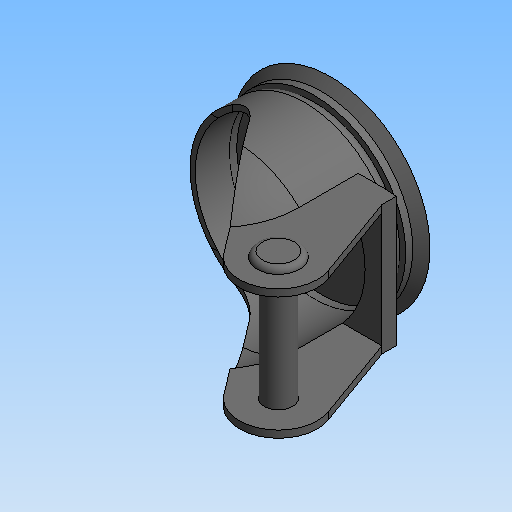
# Autodesk Inventor part: BODY-HSMCS50
Saved by Autodesk Inventor 2020 (Build 240168000, 168)
## iProperties
Part Number: BODY-HSMCS50
Material: 一般
Catalog Web Link: www.cadenas.de
Description: HSMC-BODY-Casters for Aluminum Frames-Corner Angle Type
Vendor: MISUMI
Document SubType Name: Modeling
Designer: partserver
Manufacturer: MISUMI
Mass: 15.0578 g
Surface Area: 150.838 cm^2
Volume: 15.0578 cm^3
Density: 1 g/cm^3
Appearance: PSOLRGB-128-128-128
Category: PARTsolutions
Company: MISUMI
PSOL_IDENT_0: {$CADENAS_DATA\23d-libs\misumi\metric\39_accessories_for_al_extrusions\hsmc.prj},167 {VTYP=3D},{NB=B
PSOL_IDENT_1: ODY-HSMCS50},{LINA=BODY-HSMCS50},{NN=HSMC-BODY},{DATE=30.06.2021 13:18:54},{GEOMDATE=20.12.2007 07:3
PSOL_IDENT_2: 1:00},{VERSION=},{LINEID=60},{WBVAR=},{WBNUMERIC=}  {NB=BODY-HSMCS50},{LINA=BODY-HSMCS50},{KT=DUMMY}
PSOL_IDENT_3: ,{D=50},{TYPE=HSMCS},{AF=HFS5-2020},{H=70},{B=28},{DD=5.3},{E=27},{DD1=34.703},{DD2=2.800},{DD3=56.0
PSOL_IDENT_4: 00},{DD4=29.936},{DD5=42.809},{DD6=12.029},{DD7=37},{DD8=27.000},{DD9=22.000},{DD10=45.000},{DD11=30
PSOL_IDENT_5: .233},{PN=BODY-HSMCS50}
NB: BODY-HSMCS50
NN: HSMC-BODY
NT: Casters for Aluminum Frames-Corner Angle Type
NBSYN: $PN.
LINA: BODY-HSMCS50
CATALOG: Misumi
D: 50
TYPE: HSMCS
AF: HFS5-2020
H: 70
B: 28
DD: 5.3
E: 27
DD1: 34.703
DD2: 2.8
DD3: 56
DD4: 29.936
DD5: 42.809
DD6: 12.029
DD7: 37
DD8: 27
DD9: 22
DD10: 45
DD11: 30.233
SUPPLIER: MISUMI
ARTICLENO: BODY-HSMCS50
BOMINFO: BODY-HSMCS50
CREATOR: CADENAS GmbH
Title: BODY-HSMCS50
Author: Cadenas PARTsolutions
Comments: Casters for Aluminum Frames-Corner Angle Type
Autodesk Inventor part; units mm, degrees
sketch "Sketch_1" plane through (0, 0, 0) normal (1, 0, 0) x (0, 1, 0)
  line L0 (-56, 0) -> (0, 0)
  line L1 (-3.2, 0) -> (-3.2, -28.075)
  line L2 (-3.2, -28.075) -> (-5.8, -25.22)
  line L3 (-5.8, -25.22) -> (-5.8, -25.7879)
  line L4 (-5.8, -25.7879) -> (-7.8, -25.7879)
  line L5 (-7.8, -25.7879) -> (-7.8, -24.1)
  arc A0 (-10.6, -25.5) -> (-7.8, -24.1) centre (-10.6, -22) ccw
  line L6 (-10.6, -25.5) -> (-29.936, -25.5)
  arc A1 (-51.0993, -18.3) -> (-29.936, -25.5) centre (-29.936, 9.203) ccw
  line L7 (-51.0993, -18.3) -> (-56, -18.3)
  line L8 (-56, -18.3) -> (-56, 0)
  line L9 (-56, 0) -> (-3.2, 0)
  constraints: 20 end point, 4 point on circle, 2 centre point
revolve "Revolution1" add sketch "Sketch_1" angle 360 about axis through (0, -56, 0) along (0, -1, 0)
sketch "Sketch_2" plane through (0, 0, 0) normal (0, 0, 1) x (1, 0, 0)
  line L0 (-50, -13.191) -> (-21.7584, -56)
  line L1 (-21.7584, -56) -> (-17.7584, -56)
  line L2 (-17.7584, -56) -> (-17.7584, -13.191)
  line L3 (-17.7584, -13.191) -> (-50, -13.191)
  constraints: 8 end point
extrude "Extrusion1" cut sketch "Sketch_2" along normal mid plane 56
sketch "Sketch_3" plane through (0, 0, 0) normal (0, 0, 1) x (1, 0, 0)
  line L0 (-150, -150) -> (150, -150)
  line L1 (150, -150) -> (150, 150)
  line L2 (150, 150) -> (-150, 150)
  line L3 (-150, 150) -> (-150, -150)
  arc A0 (-37.3451, -41.2613) -> (-18.215, -51.6199) centre (-27, -45) ccw
  line L4 (-18.215, -51.6199) -> (3.8878, -22.2883)
  arc A1 (13.4715, -17.51) -> (3.8878, -22.2883) centre (13.4715, -29.51) ccw
  line L5 (13.4715, -17.51) -> (27.5, -17.51)
  line L6 (27.5, -17.51) -> (27.5, 0)
  line L7 (27.5, 0) -> (-28.7615, 0)
  line L8 (-28.7615, 0) -> (-28.7615, -17.51)
  line L9 (-28.7615, -17.51) -> (-37.3451, -41.2613)
  constraints: 20 end point, 4 point on circle, 2 centre point
sketch "Sketch_5" plane through (-17.7584, 0, 0) normal (1, 0, 0) x (0, 0, -1)
  line L0 (-18.3, -56) -> (-16.3, -56)
  line L1 (-16.3, -56) -> (-16.3, -17.501)
  line L2 (-16.3, -17.501) -> (16.3, -17.501)
  line L3 (16.3, -17.501) -> (16.3, -56)
  line L4 (16.3, -56) -> (18.3, -56)
  line L5 (18.3, -56) -> (18.3, -13.191)
  line L6 (18.3, -13.191) -> (-18.3, -13.191)
  line L7 (-18.3, -13.191) -> (-18.3, -56)
  constraints: 16 end point
extrude "Extrusion2" add sketch "Sketch_5" along normal mid plane 44
extrude "Extrusion3" cut sketch "Sketch_3" along normal mid plane 100
sketch "Sketch_4" plane through (0, -5.8, 0) normal (0, 1, 0) x (1, 0, 0)
  circle A0 centre (0, 0) radius 24
  constraints: 1 centre point
extrude "Extrusion4" cut sketch "Sketch_4" against normal blind 24.076
sketch "Sketch_6" plane through (0, 0, 0) normal (1, 0, 0) x (0, 1, 0)
  line L0 (-56, 0) -> (0, 0)
  line L1 (-29.6366, 0) -> (-29.6366, -24)
  line L2 (-29.6366, -24) -> (-29.936, -24)
  arc A0 (-51.0993, -16.8) -> (-29.936, -24) centre (-29.936, 10.703) ccw
  line L3 (-51.0993, -16.8) -> (-51.0993, 0)
  line L4 (-51.0993, 0) -> (-29.6366, 0)
  constraints: 10 end point, 2 point on circle, 1 centre point
revolve "Revolution2" cut sketch "Sketch_6" angle 360 about axis through (0, -56, 0) along (0, -1, 0)
sketch "Sketch_7" plane through (0, 0, 0) normal (1, 0, 0) x (0, 1, 0)
  line L0 (-56, 16.3) -> (-56, -16.3)
  line L1 (-56, -16.3) -> (-17.501, -16.3)
  line L2 (-17.501, -16.3) -> (-17.501, 16.3)
  line L3 (-17.501, 16.3) -> (-56, 16.3)
  constraints: 8 end point
extrude "Extrusion5" cut sketch "Sketch_7" along normal mid plane 116
sketch "Sketch_8" plane through (0, 0, 0) normal (0, 0, 1) x (1, 0, 0)
  line L0 (-50, -15.3345) -> (-25.5, -13.191)
  line L1 (-25.5, -13.191) -> (-50, -13.191)
  line L2 (-50, -13.191) -> (-50, -15.3345)
  constraints: 6 end point
extrude "Extrusion6" cut sketch "Sketch_8" along normal mid plane 116
sketch "Sketch_9" plane through (0, 0, 0) normal (0, 0, 1) x (1, 0, 0)
  circle A0 centre (-27, -45) radius 4
  constraints: 1 centre point
extrude "Extrusion7" add sketch "Sketch_9" along normal mid plane 36.6
sketch "Sketch_10" plane through (-27, 0, 0) normal (1, 0, 0) x (0, 0, -1)
  line L0 (19.8, -45) -> (18.3, -45)
  line L1 (18.3, -45) -> (18.3, -39)
  arc A0 (19.8, -40.5) -> (18.3, -39) centre (18.3, -40.5) ccw
  line L2 (19.8, -40.5) -> (19.8, -45)
  line L3 (19.8, -45) -> (18.3, -45)
  constraints: 8 end point, 2 point on circle, 1 centre point
revolve "Revolution3" add sketch "Sketch_10" angle 360 about axis through (-27, -45, -19.8) along (0, 0, -1)
ref_plane "body_to_dummy_XY" through (0, 0, 0) normal (0, -1, 0) x (1, 0, 0)
ref_plane "body_to_dummy_YZ" through (0, 0, 0) normal (1, 0, 0) x (0, 0, 1)
ref_plane "body_to_dummy_ZX" through (0, 0, 0) normal (0, 0, 1) x (0, -1, 0)
ref_plane "body_to_stopper_left_XY" through (-27, -45, -18.3) normal (0, 0, -1) x (1, 0, 0)
ref_plane "body_to_stopper_left_YZ" through (-27, -45, -18.3) normal (1, 0, 0) x (0, -1, 0)
ref_plane "body_to_stopper_left_ZX" through (-27, -45, -18.3) normal (0, -1, 0) x (0, 0, -1)
ref_plane "body_to_stopper_right_XY" through (-27, -45, 18.3) normal (0, 0, 1) x (1, 0, 0)
ref_plane "body_to_stopper_right_YZ" through (-27, -45, 18.3) normal (1, 0, 0) x (0, 1, 0)
ref_plane "body_to_stopper_right_ZX" through (-27, -45, 18.3) normal (0, 1, 0) x (0, 0, 1)
ref_plane "body_to_swivel_XY" through (0, -3.2, 0) normal (0, -1, 0) x (1, 0, 0)
ref_plane "body_to_swivel_YZ" through (0, -3.2, 0) normal (1, 0, 0) x (0, 0, 1)
ref_plane "body_to_swivel_ZX" through (0, -3.2, 0) normal (0, 0, 1) x (0, -1, 0)
ref_plane "body_to_wheel_XY" through (-27, -45, 0) normal (0, 0, 1) x (1, 0, 0)
ref_plane "body_to_wheel_YZ" through (-27, -45, 0) normal (1, 0, 0) x (0, 1, 0)
ref_plane "body_to_wheel_ZX" through (-27, -45, 0) normal (0, 1, 0) x (0, 0, 1)
body "Solid1"
